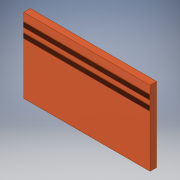
# Autodesk Inventor part: PowerRail
Saved by Autodesk Inventor 2019 (Build 230136000, 136)
## iProperties
Created: 2018-10-16
Part Number: PowerRail
Material: Generisch
Document SubType Name: Modeling
Designer: janbe
Density: 1 g/cm^3
Appearance: Glatt - Hellorange
Author: janbe
Autodesk Inventor part; units mm, degrees
ref_plane "YZ Plane" through (0, 0, 0) normal (1, 0, 0) x (0, 1, 0)
ref_plane "XZ Plane" through (0, 0, 0) normal (0, 1, 0) x (-1, 0, 0)
ref_plane "XY Plane" through (0, 0, 0) normal (0, 0, 1) x (1, 0, 0)
sketch "Skizze1" plane through (0, 0, 0) normal (0, 0, 1) x (1, 0, 0)
  line L0 (0, 0) -> (33, 0)
  line L1 (33, 0) -> (33, -19.5)
  line L2 (33, -19.5) -> (0, -19.5)
  line L3 (0, -19.5) -> (0, 0)
  dimension "d0" = 33
  dimension "d1" = 19.5
  constraints: 8 end point, 2 parallel, 1 horizontal, 1 perpendicular
  measures "d0" distance of L1.end L2.end
  measures "d1" distance of L0.end L1.end
extrude "Extrusion1" add sketch "Skizze1" along normal blind 1.7
sketch "Skizze2" plane through (0, 0, 1.7) normal (0, 0, 1) x (1, 0, 0)
  line L0 (33, 0) -> (0, 0) projected
  line L1 (0, 0) -> (0, -19.5) projected
  line L2 (0, -19.5) -> (33, -19.5) projected
  line L3 (33, -19.5) -> (33, 0) projected
  line L4 (0, 0) -> (0, -19.5) projected
  line L5 (33, 0) -> (33, -19.5) projected
  line L6 (0, -2.15) -> (33, -2.15)
  line L7 (33, -2.15) -> (33, -3.35)
  line L8 (33, -3.35) -> (0, -3.35)
  line L9 (0, -3.35) -> (0, -2.15)
  line L10 (33, -5.85) -> (0, -5.85)
  line L11 (0, -5.85) -> (0, -4.65)
  line L12 (0, -4.65) -> (33, -4.65)
  line L13 (33, -4.65) -> (33, -5.85)
  line L14 (0, -3.35) -> (33, -3.35)
  line L15 (33, -3.35) -> (33, -2.15)
  line L16 (33, -2.15) -> (0, -2.15)
  line L17 (0, -2.15) -> (0, -3.35)
  line L18 (33, -4.65) -> (0, -4.65)
  line L19 (0, -4.65) -> (0, -5.85)
  line L20 (0, -5.85) -> (33, -5.85)
  line L21 (33, -5.85) -> (33, -4.65)
  dimension "d10" = 1.2
  dimension "d11" = 1.2
  dimension "d12" = 1.3
  constraints: 32 end point, 8 parallel, 4 horizontal, 4 perpendicular, 4 point on line
  measures "d10" distance of L12.end L10.start
  measures "d11" distance between parallel lines of L8 L6
  measures "d12" distance between parallel lines of L12 L8
extrude "Extrusion2" add sketch "Skizze2" along normal blind 0.1 contours L3 L8 L1 L6 | L3 L10 L1 L12
sketch "Skizze4" plane through (0, 0, 1.7) normal (0, 0, 1) x (1, 0, 0)
  line L0 (429, -5.85) -> (0, -5.85) projected
  line L1 (0, -5.85) -> (0, -20) projected
  line L2 (0, -20) -> (429, -20) projected
  line L3 (429, -20) -> (429, -5.85) projected
  line L4 (0, -20) -> (-50, -20)
  line L5 (-50, -20) -> (-50, 20)
  line L6 (-50, 20) -> (0, 20)
  line L7 (0, 20) -> (0, -20)
  line L8 (23.5, 20) -> (11.5, 20) projected
  point P0 (0, 0)
  dimension "d19" = 50
  constraints: 8 end point, 2 parallel, 1 collinear, 1 horizontal, 1 perpendicular
  measures "d19" distance of L5.end L6.end
sketch "Skizze5" plane through (0, 0, 1.7) normal (0, 0, 1) x (1, 0, 0)
  circle A0 centre (50.5, 14) radius 1.5 projected
  circle A1 centre (83.5, 14) radius 1.5 projected
  circle A2 centre (116.5, 14) radius 1.5 projected
  circle A3 centre (149.5, 14) radius 1.5 projected
  circle A4 centre (182.5, 14) radius 1.5 projected
  circle A5 centre (215.5, 14) radius 1.5 projected
  circle A6 centre (248.5, 14) radius 1.5 projected
  circle A7 centre (281.5, 14) radius 1.5 projected
  circle A8 centre (314.5, 14) radius 1.5 projected
  circle A9 centre (347.5, 14) radius 1.5 projected
  circle A10 centre (380.5, 14) radius 1.5 projected
  circle A11 centre (413.5, 14) radius 1.5 projected
  circle A12 centre (17.5, 14) radius 1.5 projected
  line L0 (0, -2.15) -> (429, -2.15) projected
  line L1 (429, -2.15) -> (429, 0) projected
  line L2 (429, 0) -> (419.5, 0) projected
  line L3 (419.5, 0) -> (419.5, 20) projected
  line L4 (419.5, 20) -> (407.5, 20) projected
  line L5 (407.5, 20) -> (407.5, 0) projected
  line L6 (407.5, 0) -> (386.5, 0) projected
  line L7 (386.5, 0) -> (386.5, 20) projected
  line L8 (386.5, 20) -> (374.5, 20) projected
  line L9 (374.5, 20) -> (374.5, 0) projected
  line L10 (374.5, 0) -> (353.5, 0) projected
  line L11 (353.5, 0) -> (353.5, 20) projected
  line L12 (353.5, 20) -> (341.5, 20) projected
  line L13 (341.5, 20) -> (341.5, 0) projected
  line L14 (341.5, 0) -> (320.5, 0) projected
  line L15 (320.5, 0) -> (320.5, 20) projected
  line L16 (320.5, 20) -> (308.5, 20) projected
  line L17 (308.5, 20) -> (308.5, 0) projected
  line L18 (308.5, 0) -> (287.5, 0) projected
  line L19 (287.5, 0) -> (287.5, 20) projected
  line L20 (287.5, 20) -> (275.5, 20) projected
  line L21 (275.5, 20) -> (275.5, 0) projected
  line L22 (275.5, 0) -> (254.5, 0) projected
  line L23 (254.5, 0) -> (254.5, 20) projected
  line L24 (254.5, 20) -> (242.5, 20) projected
  line L25 (242.5, 20) -> (242.5, 0) projected
  line L26 (242.5, 0) -> (221.5, 0) projected
  line L27 (221.5, 0) -> (221.5, 20) projected
  line L28 (221.5, 20) -> (209.5, 20) projected
  line L29 (209.5, 20) -> (209.5, 0) projected
  line L30 (209.5, 0) -> (188.5, 0) projected
  line L31 (188.5, 0) -> (188.5, 20) projected
  line L32 (188.5, 20) -> (176.5, 20) projected
  line L33 (176.5, 20) -> (176.5, 0) projected
  line L34 (176.5, 0) -> (155.5, 0) projected
  line L35 (155.5, 0) -> (155.5, 20) projected
  line L36 (155.5, 20) -> (143.5, 20) projected
  line L37 (143.5, 20) -> (143.5, 0) projected
  line L38 (143.5, 0) -> (122.5, 0) projected
  line L39 (122.5, 0) -> (122.5, 20) projected
  line L40 (122.5, 20) -> (110.5, 20) projected
  line L41 (110.5, 20) -> (110.5, 0) projected
  line L42 (110.5, 0) -> (89.5, 0) projected
  line L43 (89.5, 0) -> (89.5, 20) projected
  line L44 (89.5, 20) -> (77.5, 20) projected
  line L45 (77.5, 20) -> (77.5, 0) projected
  line L46 (77.5, 0) -> (56.5, 0) projected
  line L47 (56.5, 0) -> (56.5, 20) projected
  line L48 (56.5, 20) -> (44.5, 20) projected
  line L49 (44.5, 20) -> (44.5, 0) projected
  line L50 (44.5, 0) -> (23.5, 0) projected
  line L51 (23.5, 0) -> (23.5, 20) projected
  line L52 (23.5, 20) -> (11.5, 20) projected
  line L53 (11.5, 20) -> (11.5, 0) projected
  line L54 (11.5, 0) -> (0, 0) projected
  line L55 (0, 0) -> (0, 20) projected
  line L56 (0, 20) -> (-50, 20) projected
  line L57 (-50, 20) -> (-50, -20) projected
  line L58 (-50, -20) -> (429, -20) projected
  line L59 (429, -20) -> (429, -5.85) projected
  line L60 (429, -5.85) -> (0, -5.85) projected
  line L61 (0, -4.65) -> (0, -5.85) projected
  line L62 (0, -4.65) -> (429, -4.65) projected
  line L63 (429, -4.65) -> (429, -3.35) projected
  line L64 (429, -3.35) -> (0, -3.35) projected
  line L65 (0, -2.15) -> (0, -3.35) projected
  line L66 (-38.9172, -16.707) -> (-48.9487, -16.707)
  line L67 (-48.9487, -16.707) -> (-48.9487, -8.753)
  line L68 (-48.9487, -8.753) -> (-38.9172, -8.753)
  line L69 (-38.9172, -8.753) -> (-38.9172, -16.707)
  line L70 (-40.6386, -6.9723) -> (-48.9487, -6.9723)
  line L71 (-48.9487, -6.9723) -> (-48.9487, -2.75)
  line L72 (-48.9487, -2.75) -> (-40.6386, -2.75)
  line L73 (-40.6386, -2.75) -> (-40.6386, -6.9723)
  constraints: 16 end point, 4 parallel, 2 horizontal, 2 perpendicular, 1 point on line
sketch "Skizze6" plane through (0, 0, 1.7) normal (0, 0, 1) x (1, 0, 0)
  circle A0 centre (-40.9672, 3.5952) radius 2
  point P0 (0, 0)
  dimension "d25" = 4
  dimension "d29" = 20
  dimension "d30" = 1.3
  dimension "d31" = 1.2
  dimension "d32" = 1.2
  dimension "d33" = 2.15
  constraints: 1 centre point
